Autodesk Fusion 360 part; units mm, degrees
(part 5 of 5)
  spline S779 degree 3 poles (56.8712, -40.9571) (57.9641, -40.6744) (58.6812, -39.7955) (58.4742, -38.995) knots 2 2 2 2 3 3 3 3
  spline S780 degree 3 poles (58.4742, -38.995) (58.2669, -38.1945) (57.107, -37.3653) (56.0145, -37.6481) knots 3 3 3 3 4 4 4 4
  spline S781 degree 3 poles (53.4083, -36.7351) (55.0489, -34.3649) (57.5041, -35.5915) (57.608, -35.6452) knots 0 0 0 0 1 1 1 1
  spline S782 degree 3 poles (57.608, -35.6452) (57.7123, -35.6985) (57.8408, -35.6577) (57.8949, -35.5532) knots 1 1 1 1 2 2 2 2
  spline S783 degree 3 poles (57.8949, -35.5532) (57.9491, -35.4491) (57.9083, -35.3203) (57.8038, -35.2666) knots 2 2 2 2 3 3 3 3
  spline S784 degree 3 poles (57.8038, -35.2666) (57.7848, -35.2566) (56.5123, -34.6152) (55.1157, -34.9771) knots 3 3 3 3 4 4 4 4
  spline S785 degree 3 poles (55.1157, -34.9771) (54.413, -35.1591) (53.6789, -35.5952) (53.0574, -36.4928) knots 4 4 4 4 5 5 5 5
  spline S786 degree 3 poles (53.0574, -36.4928) (52.9905, -36.5894) (53.0148, -36.7222) (53.1116, -36.7893) knots 5 5 5 5 6 6 6 6
  spline S787 degree 3 poles (53.1116, -36.7893) (53.2082, -36.8564) (53.3411, -36.8322) (53.4083, -36.7351) knots 6 6 6 6 7 7 7 7
sketch "Sketch12" plane through (0, 0, 42.25) normal (0, 0, 1) x (1, 0, 0)
  line L0 (82, 45.25) -> (82, 75.25)
  line L1 (82, 125.25) -> (82, 155.25)
  line L2 (82, 205.25) -> (82, 235.25)
  line L3 (-2, 44.25) -> (82, 44.25)
  line L4 (-2, 44.25) -> (84, 44.25)
  line L5 (84, 244) -> (-2, 244)
  line L6 (82, 235.25) -> (84, 235.25) construction
  line L7 (82, 205.25) -> (84, 205.25) construction
  line L8 (82, 155.25) -> (84, 155.25) construction
  line L9 (82, 125.25) -> (84, 125.25) construction
  line L10 (82, 75.25) -> (84, 75.25) construction
  line L11 (82, 45.25) -> (84, 45.25) construction
  line L12 (84, 45.25) -> (87, 45.25)
  line L13 (87, 45.25) -> (87, 75.25)
  line L14 (87, 75.25) -> (84, 75.25)
  line L15 (84, 44.25) -> (84, 45.25)
  line L16 (84, 125.25) -> (87, 125.25)
  line L17 (87, 125.25) -> (87, 155.25)
  line L18 (87, 155.25) -> (84, 155.25)
  line L19 (84, 75.25) -> (84, 125.25)
  line L20 (84, 205.25) -> (87, 205.25)
  line L21 (87, 205.25) -> (87, 235.25)
  line L22 (87, 235.25) -> (84, 235.25)
  line L23 (84, 155.25) -> (84, 205.25)
  line L24 (84, 235.25) -> (84, 244)
  line L25 (41, 19.25) -> (41, 69.25) construction
  line L26 (-5, 235.25) -> (-2, 235.25)
  line L27 (-5, 205.25) -> (-5, 235.25)
  line L28 (-2, 205.25) -> (-5, 205.25)
  line L29 (-5, 155.25) -> (-2, 155.25)
  line L30 (-5, 125.25) -> (-5, 155.25)
  line L31 (-2, 125.25) -> (-5, 125.25)
  line L32 (-5, 75.25) -> (-2, 75.25)
  line L33 (-5, 45.25) -> (-5, 75.25)
  line L34 (-2, 45.25) -> (-5, 45.25)
  line L35 (-2, 45.25) -> (-2, 44.25)
  line L36 (-2, 125.25) -> (-2, 75.25)
  line L37 (-2, 244) -> (-2, 235.25)
  line L38 (-2, 205.25) -> (-2, 155.25)
  point P0 (40, 244)
  point P1 (40, 244)
  point P2 (41, 44.25)
  dimension "d141" = 86
  dimension "d142" = 3
  dimension "d143" = 30
  dimension "d144" = 3
  dimension "d145" = 30
  dimension "d146" = 3
  dimension "d147" = 30
  dimension "d148" = 50
  constraint horizontal L4
  constraint vertical L15
  constraint horizontal L5
  constraint vertical L37
  constraint coincident L3.start L4.start
  constraint coincident L5 P1
  constraint coincident L2.end L6.start
  constraint perpendicular L6 L24
  constraint coincident L2.start L7.start
  constraint perpendicular L7 L23
  constraint coincident L1.end L8.start
  constraint perpendicular L8 L23
  constraint coincident L1.start L9.start
  constraint perpendicular L9 L19
  constraint coincident L0.end L10.start
  constraint perpendicular L10 L19
  constraint coincident L0.start L11.start
  constraint perpendicular L11 L15
  constraint horizontal L12
  constraint vertical L13
  constraint horizontal L14
  constraint collinear L15 L19
  constraint horizontal L16
  constraint vertical L17
  constraint horizontal L18
  constraint collinear L19 L23
  constraint horizontal L20
  constraint vertical L21
  constraint horizontal L22
  constraint collinear L23 L24
  constraint coincident P1 P0
  constraint midpoint L25 P2
  constraint coincident L4 P2
  constraint perpendicular L3 L25
  constraint symmetric L7.end L25 L28.start
  constraint symmetric L9.end L25 L31.start
  constraint symmetric L11.end L25 L34.start
  constraint symmetric L12.end L25 L33.start
  constraint symmetric L13.end L25 L32.start
  constraint symmetric L10.end L25 L32.end
  constraint symmetric L16.end L25 L30.start
  constraint symmetric L17.end L25 L29.start
  constraint symmetric L8.end L25 L29.end
  constraint symmetric L20.end L25 L27.start
  constraint symmetric L21.end L25 L26.start
  constraint symmetric L6.end L25 L26.end
  constraint collinear L35 L36
  constraint collinear L36 L38
  constraint collinear L37 L38
  measures "d141" distance of L3.start L4.end
  measures "d142" distance of L11.end L12.end
  measures "d143" distance of L11.end L10.end
  measures "d144" distance of L9.end L16.end
  measures "d145" distance of L9.end L8.end
  measures "d146" distance of L7.end L20.end
  measures "d147" distance of L7.end L6.end
  measures "d148" distance of L25.start L25.end
equation "stepper_length = 40 mm"
equation "stepper_width = 42.25 mm"
equation "stepper_height = stepper_width"
equation "wall_thickness = 2 mm"
equation "stepper_screw_diameter = 4 mm"
equation "base_screw_diameter = 5 mm"
equation "base_thickness = 2 mm"
equation "base_flap_size = 15 mm"
equation "d9 = 2 * stepper_length"
equation "d10 = stepper_width"
equation "d11 = wall_thickness"
equation "d12 = wall_thickness"
equation "d13 = 2 * stepper_length + 2 * wall_thickness"
equation "d14 = stepper_width + 2 * wall_thickness"
equation "d15 = stepper_length * 2 + 2 * wall_thickness"
equation "d16 = base_flap_size"
equation "d17 = base_screw_diameter"
equation "d18 = base_screw_diameter"
equation "d19 = stepper_height"
equation "d21 = -base_thickness"
equation "side_to_screw = 6 mm"
equation "d24 = side_to_screw"
equation "d25 = side_to_screw"
equation "d26 = stepper_screw_diameter"
equation "d27 = stepper_width / 2"
equation "d28 = stepper_height / 2"
equation "stepper_circle_diameter = 22 mm"
equation "d32 = stepper_circle_diameter"
equation "d33 = stepper_height / 2"
equation "material_thickness = 3 mm"
equation "d40 = material_thickness + wall_thickness + motor_cap_thickness"
equation "d41 = material_thickness + wall_thickness + motor_cap_thickness"
equation "car_base_width = material_thickness * 2 + 2 * wall_thickness + stepper_length * 2 + 2 * motor_cap_thickness"
equation "car_base_length = 250 mm"
equation "d44 = car_base_width"
equation "d45 = car_base_length"
equation "front_to_wheel = 20 mm"
equation "d47 = car_base_width / 2"
equation "d48 = front_to_wheel"
equation "small_wheel_diameter = 30 mm"
equation "d50 = small_wheel_diameter"
equation "front_wheel_to_screw = 2 mm"
equation "d52 = front_wheel_to_screw"
equation "d53 = base_screw_diameter"
equation "d55 = base_screw_diameter"
equation "d56 = base_screw_diameter"
equation "d57 = base_screw_diameter"
equation "finger_length = 10 mm"
equation "d60 = finger_length"
equation "d61 = material_thickness"
equation "d62 = finger_length"
equation "d63 = finger_length"
equation "d64 = material_thickness"
equation "d65 = finger_length"
equation "d66 = stepper_height"
equation "motor_cap_thickness = 1 mm"
equation "d68 = motor_cap_thickness"
equation "d69 = motor_cap_thickness"
equation "d70 = motor_cap_thickness"
equation "d71 = motor_cap_thickness"
equation "d72 = motor_cap_thickness"
equation "d73 = motor_cap_thickness"
equation "d74 = motor_cap_thickness"
equation "d75 = motor_cap_thickness"
equation "motor_cap_bottom_height = 3 mm"
equation "motor_cap_top_height = 1 mm"
equation "d78 = -motor_cap_bottom_height"
equation "d80 = -motor_cap_bottom_height"
equation "cap_hole_width = 30 mm"
equation "cap_hole_height = 20 mm"
equation "d86 = cap_hole_width"
equation "d87 = cap_hole_height"
equation "d90 = motor_cap_top_height"
equation "d92 = finger_length"
equation "d93 = material_thickness"
equation "d94 = finger_length"
equation "d95 = finger_length"
equation "d96 = finger_length"
equation "d97 = material_thickness"
equation "d98 = finger_length"
equation "d99 = finger_length"
equation "d100 = material_thickness"
equation "car_height = 90 mm"
equation "base_to_layer_1 = material_thickness + stepper_height - motor_cap_bottom_height"
equation "d103 = base_thickness"
equation "d104 = car_base_length"
equation "d105 = car_height"
equation "slit_length = 30 mm"
equation "d107 = slit_length"
equation "d108 = material_thickness"
equation "d113 = stepper_circle_diameter"
equation "d114 = finger_length"
equation "d115 = material_thickness"
equation "d116 = finger_length"
equation "d117 = material_thickness"
equation "d118 = finger_length"
equation "d119 = material_thickness"
equation "d120 = finger_length"
equation "d121 = material_thickness"
equation "d122 = finger_length"
equation "d123 = finger_length"
equation "d124 = material_thickness"
equation "d125 = finger_length"
equation "d126 = material_thickness"
equation "d127 = material_thickness"
equation "d128 = car_base_width"
equation "d129 = finger_length"
equation "d130 = material_thickness"
equation "d131 = finger_length"
equation "d132 = material_thickness"
equation "d133 = finger_length"
equation "d134 = material_thickness"
equation "d135 = finger_length"
equation "d136 = material_thickness"
equation "d137 = material_thickness"
equation "d138 = finger_length"
equation "d139 = material_thickness"
equation "d140 = finger_length"
equation "d141 = car_base_width - 2 * material_thickness"
equation "d142 = material_thickness"
equation "d143 = slit_length"
equation "d144 = material_thickness"
equation "d145 = slit_length"
equation "d146 = material_thickness"
equation "d147 = slit_length"
